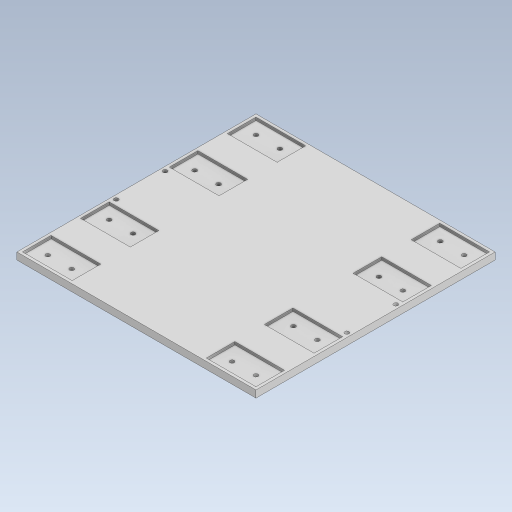
# Autodesk Inventor part: Casis
Saved by Autodesk Inventor 2023.5 (Build 275446000, 446)
## iProperties
Created: 2025-09-05
Part Number: Casis
Material: Generic
Document SubType Name: Modeling
Designer: Guntur
Density: 1 g/cm^3
Appearance: Default
Author: Guntur
Autodesk Inventor part; units mm, degrees
ref_plane "YZ Plane" through (0, 0, 0) normal (1, 0, 0) x (0, 1, 0)
ref_plane "XZ Plane" through (0, 0, 0) normal (0, 1, 0) x (-1, 0, 0)
ref_plane "XY Plane" through (0, 0, 0) normal (0, 0, 1) x (1, 0, 0)
sketch "Sketch2" plane through (0, 0, 0) normal (0, 1, 0) x (-1, 0, 0)
  line L0 (85, 85) -> (-85, 85)
  line L1 (-85, 85) -> (-85, -85)
  line L2 (-85, -85) -> (85, -85)
  line L3 (85, -85) -> (85, 85)
  line L4 (85, 0) -> (-85, 0) construction
  line L5 (0, 85) -> (0, -85) construction
  line L6 (83, 83) -> (47.7, 83)
  line L7 (47.7, 83) -> (47.7, 62.7)
  line L8 (47.7, 62.7) -> (83, 62.7)
  line L9 (83, 62.7) -> (83, 83)
  line L10 (83, 41.7) -> (47.7, 41.7)
  line L11 (47.7, 41.7) -> (47.7, 21.4)
  line L12 (47.7, 21.4) -> (83, 21.4)
  line L13 (83, 21.4) -> (83, 41.7)
  circle A0 centre (74, 74) radius 1.5
  circle A1 centre (57, 74) radius 1.5
  circle A2 centre (74, 30.4) radius 1.5
  circle A3 centre (57, 30.4) radius 1.5
  line L14 (83, -83) -> (47.7, -83)
  line L15 (47.7, -83) -> (47.7, -62.7)
  line L16 (47.7, -62.7) -> (83, -62.7)
  line L17 (83, -62.7) -> (83, -83)
  line L18 (83, -41.7) -> (47.7, -41.7)
  line L19 (47.7, -41.7) -> (47.7, -21.4)
  line L20 (47.7, -21.4) -> (83, -21.4)
  line L21 (83, -21.4) -> (83, -41.7)
  circle A4 centre (74, -74) radius 1.5
  circle A5 centre (57, -74) radius 1.5
  circle A6 centre (74, -30.4) radius 1.5
  circle A7 centre (57, -30.4) radius 1.5
  line L22 (-83, 83) -> (-47.7, 83)
  line L23 (-47.7, 83) -> (-47.7, 62.7)
  line L24 (-47.7, 62.7) -> (-83, 62.7)
  line L25 (-83, 62.7) -> (-83, 83)
  line L26 (-83, 41.7) -> (-47.7, 41.7)
  line L27 (-47.7, 41.7) -> (-47.7, 21.4)
  line L28 (-47.7, 21.4) -> (-83, 21.4)
  line L29 (-83, 21.4) -> (-83, 41.7)
  circle A8 centre (-74, 74) radius 1.5
  circle A9 centre (-57, 74) radius 1.5
  circle A10 centre (-74, 30.4) radius 1.5
  circle A11 centre (-57, 30.4) radius 1.5
  line L30 (-47.7, -62.7) -> (-83, -62.7)
  circle A12 centre (-57, -74) radius 1.5
  circle A13 centre (-74, -74) radius 1.5
  line L31 (-47.7, -83) -> (-47.7, -62.7)
  line L32 (-83, -83) -> (-47.7, -83)
  line L33 (-83, -62.7) -> (-83, -83)
  line L34 (-83, -41.7) -> (-47.7, -41.7)
  circle A14 centre (-57, -30.4) radius 1.5
  circle A15 centre (-74, -30.4) radius 1.5
  line L35 (-83, -21.4) -> (-83, -41.7)
  line L36 (-47.7, -41.7) -> (-47.7, -21.4)
  line L37 (-47.7, -21.4) -> (-83, -21.4)
  circle A16 centre (-82, 17.4) radius 1.5
  circle A17 centre (-82, -17.4) radius 1.5
  circle A18 centre (82, 17.4) radius 1.5
  circle A19 centre (82, -17.4) radius 1.5
  point P0 (0, 0)
  point P1 (83, 72.85)
  point P2 (65.35, 83)
  point P3 (83, -72.85)
  point P4 (65.35, -83)
  point P5 (-83, 72.85)
  point P6 (-65.35, 83)
  point P7 (-83, -72.85)
  point P8 (-65.35, -83)
  dimension "d17" = 170
  dimension "d18" = 170
  dimension "d19" = 35.3
  dimension "d20" = 20.3
  dimension "d21" = 2
  dimension "d22" = 2
  dimension "d23" = 20.3
  dimension "d24" = 21
  dimension "d25" = 3
  dimension "d26" = 9
  dimension "d27" = 9
  dimension "d28" = 3
  dimension "d29" = 17
  dimension "d30" = 3
  dimension "d31" = 9
  dimension "d32" = 9
  dimension "d33" = 3
  dimension "d38" = 3
  dimension "d39" = 3
  dimension "d40" = 4
  dimension "d41" = 34.8
  constraints: 76 end point, 45 symmetric about line, 20 centre point, 6 midpoint, 6 parallel, 3 horizontal, 3 perpendicular, 15 other
  measures "d17" distance of L2.end L1.end
  measures "d18" distance of L1.end L0.end
  measures "d19" distance of L8.end L7.end
  measures "d20" distance of L7.end L6.end
  measures "d21" distance from line of L3 point (83, 72.85)
  measures "d22" distance from line of L0 point (65.35, 83)
  measures "d23" distance of L11.end L10.end
  measures "d24" distance between parallel lines of L10 L8
  measures "d25" diameter of A0
  measures "d26" distance from line of L9 A0.centre
  measures "d27" distance from line of L6 A0.centre
  measures "d28" diameter of A1
  measures "d29" distance of A1.centre A0.centre
  measures "d30" diameter of A2
  measures "d31" distance from line of L13 A2.centre
  measures "d32" distance from line of L12 A2.centre
  measures "d33" diameter of A3
  measures "d38" diameter of A16
  measures "d39" distance from line of L1 A16.centre
  measures "d40" distance from line of L28 A16.centre
  measures "d41" distance of A17.centre A16.centre
extrude "Extrusion3" add sketch "Sketch2" along normal blind 5 contours L3 L2 L1 L0 | A16 | A17 | A18 | A19
extrude "Extrusion4" add sketch "Sketch2" along normal blind 3 contours L9 L8 L7 L6 | L13 L12 L11 L10 | L14 L15 L16 L17 | L18 L19 L20 L21 | L22 L23 L24 L25 | L26 L27 L28 L29 | L31 L32 L33 L30 | L35 L37 L36 L34
extrude "Extrusion5" cut sketch "Sketch2" along normal blind 5 contours A16 | A17 | A18 | A19
body "Solid2"
